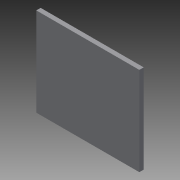
# Autodesk Inventor part: build platform
Saved by Autodesk Inventor 2013 (Build 170138000, 138)
## iProperties
Created: 2013-08-03
Part Number: build platform
Material: Generic
Document SubType Name: Modeling
Designer: employee
Density: 1 g/cm^3
Author: employee
Autodesk Inventor part; units mm, degrees
ref_plane "YZ Plane" through (0, 0, 0) normal (1, 0, 0) x (0, 1, 0)
ref_plane "XZ Plane" through (0, 0, 0) normal (0, 1, 0) x (-1, 0, 0)
ref_plane "XY Plane" through (0, 0, 0) normal (0, 0, 1) x (1, 0, 0)
sketch "Sketch1" plane through (0, 0, 0) normal (0, 0, 1) x (1, 0, 0)
  line L0 (0, 0) -> (149, 0)
  line L1 (149, 0) -> (149, 128)
  line L2 (149, 128) -> (0, 128)
  line L3 (0, 128) -> (0, 0)
  dimension "d0" = 149
  dimension "d3" = 128
  constraints: 8 end point, 2 parallel, 1 horizontal, 1 perpendicular
  measures "d0" distance of L0.start L0.end
  measures "d3" distance of L0.end L1.end
extrude "Extrusion1" add sketch "Sketch1" along normal blind 6.35
body "Solid1"
